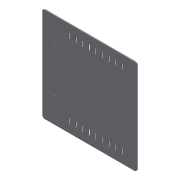
# Autodesk Inventor part: Plate A for Power Boards
Saved by Autodesk Inventor 2015 (Build 190159000, 159)
## iProperties
Created: 2015-01-10
Part Number: Plate A for Power Boards
Material: Generic
Document SubType Name: Sheet Metal
Designer: Peter
Density: 1 g/cm^3
Sheet Metal Rule: Default
Appearance: Default
Author: Peter
Autodesk Inventor part; units mm, degrees
ref_plane "YZ Plane" through (0, 0, 0) normal (1, 0, 0) x (0, 1, 0)
sketch "Sketch1" plane through (0, 0, 0) normal (0, 0, 1) x (1, 0, 0)
  line L0 (0, 0) -> (228.6, 0)
  line L1 (228.6, 0) -> (228.6, 228.6)
  line L2 (228.6, 228.6) -> (0, 228.6)
  line L3 (0, 228.6) -> (0, 0)
  dimension "d0" = 228.6
  dimension "d1" = 228.6
  measures "d0" distance of L2.end L1.end
  measures "d1" distance of L1.end L0.end
extrude "Plate1" add sketch "Sketch1" along normal blind 2.286
ref_plane "Work Plane1" through (114.3, 0, 0) normal (1, 0, 0) x (0, 0, -1)
ref_plane "Work Plane2" through (0, 114.3, 0) normal (0, 1, 0) x (1, 0, 0)
sketch "Sketch2" plane through (0, 0, 2.286) normal (0, 0, 1) x (1, 0, 0)
  circle A0 centre (29.3437, 62.0361) radius 2.667 projected
  circle A1 centre (29.3437, 166.4301) radius 2.667 projected
  circle A2 centre (211.6141, 166.4301) radius 2.667 projected
  circle A3 centre (211.6141, 62.0361) radius 2.667 projected
  circle A4 centre (29.3437, 62.0361) radius 1.5875
  circle A5 centre (29.3437, 166.4301) radius 1.5875
  circle A6 centre (211.6141, 166.4301) radius 1.5875
  circle A7 centre (211.6141, 62.0361) radius 1.5875
  dimension "x" = 3.175
  dimension "d5" = 3.175
  dimension "d6" = 3.175
  dimension "d7" = 3.175
  constraints: 4 centre point, 4 coincident
  measures "x" diameter of A4
  measures "d5" diameter of A5
  measures "d6" diameter of A6
  measures "d7" diameter of A7
sketch "Sketch3" plane through (0, 0, 2.286) normal (0, 0, 1) x (1, 0, 0)
  line L0 (0, 0) -> (0, 228.6) projected
  line L1 (228.6, 0) -> (0, 0) projected
  line L2 (228.6, 228.6) -> (228.6, 0) projected
  line L3 (0, 228.6) -> (228.6, 228.6) projected
hole "Hole1" at (29.3437, 62.0361, 2.286) direction (0, 0, -1) diameter 3.175 end through all
hole "Hole2" at (211.6141, 62.0361, 2.286) direction (0, 0, -1) diameter 3.175 end through all
hole "Hole3" at (211.6141, 166.4301, 2.286) direction (0, 0, -1) diameter 3.175 end through all
hole "Hole4" at (29.3437, 166.4301, 2.286) direction (0, 0, -1) diameter 3.175 end through all
sketch "Sketch4" plane through (0, 0, 2.286) normal (0, 0, 1) x (1, 0, 0)
  line L0 (0, 228.6) -> (228.6, 228.6) projected
  line L1 (63.5, 196.85) -> (66.675, 196.85)
  line L2 (66.675, 196.85) -> (66.675, 209.55)
  line L3 (66.675, 209.55) -> (63.5, 209.55)
  line L4 (63.5, 209.55) -> (63.5, 196.85)
  line L5 (79.375, 196.85) -> (82.55, 196.85)
  line L6 (82.55, 196.85) -> (82.55, 209.55)
  line L7 (82.55, 209.55) -> (79.375, 209.55)
  line L8 (79.375, 209.55) -> (79.375, 196.85)
  line L9 (95.25, 196.85) -> (98.425, 196.85)
  line L10 (98.425, 196.85) -> (98.425, 209.55)
  line L11 (98.425, 209.55) -> (95.25, 209.55)
  line L12 (95.25, 209.55) -> (95.25, 196.85)
  line L13 (111.125, 196.85) -> (114.3, 196.85)
  line L14 (114.3, 196.85) -> (114.3, 209.55)
  line L15 (114.3, 209.55) -> (111.125, 209.55)
  line L16 (111.125, 209.55) -> (111.125, 196.85)
  line L17 (127, 196.85) -> (130.175, 196.85)
  line L18 (130.175, 196.85) -> (130.175, 209.55)
  line L19 (130.175, 209.55) -> (127, 209.55)
  line L20 (127, 209.55) -> (127, 196.85)
  line L21 (142.875, 196.85) -> (146.05, 196.85)
  line L22 (146.05, 196.85) -> (146.05, 209.55)
  line L23 (146.05, 209.55) -> (142.875, 209.55)
  line L24 (142.875, 209.55) -> (142.875, 196.85)
  line L25 (158.75, 196.85) -> (161.925, 196.85)
  line L26 (161.925, 196.85) -> (161.925, 209.55)
  line L27 (161.925, 209.55) -> (158.75, 209.55)
  line L28 (158.75, 209.55) -> (158.75, 196.85)
  line L29 (174.625, 196.85) -> (177.8, 196.85)
  line L30 (177.8, 196.85) -> (177.8, 209.55)
  line L31 (177.8, 209.55) -> (174.625, 209.55)
  line L32 (174.625, 209.55) -> (174.625, 196.85)
  line L33 (190.5, 196.85) -> (193.675, 196.85)
  line L34 (193.675, 196.85) -> (193.675, 209.55)
  line L35 (193.675, 209.55) -> (190.5, 209.55)
  line L36 (190.5, 209.55) -> (190.5, 196.85)
  dimension "d36" = 12.7
  dimension "d37" = 3.175
  dimension "d38" = 19.05
  dimension "d39" = 63.5
  dimension "d42" = 15.875
  constraints: 72 end point, 2 horizontal, 2 parallel, 1 perpendicular, 64 other
  measures "d36" distance of L3.end L1.start
  measures "d37" distance of L1.start L1.end
  measures "d38" vertical distance of L3.end L0.start
  measures "d39" horizontal distance of L0.start L3.end
  measures "d42" distance of L3.end L8.start
extrude "Cut1" cut sketch "Sketch4" against normal blind 2.286
mirror "Mirror1" about plane through (0, 114.3, 0) normal (0, 1, 0) of "Cut1"
fillet "Corner Round1" radius 6.35 1 edges at (228.6, 228.6, 1.143)
fillet "Corner Round2" radius 6.35 3 edges at (228.6, 0, 1.143) (0, 0, 1.143) (0, 228.6, 1.143)
equation "\"d5\" = x"
equation "\"d6\" = x"
equation "\"d7\" = x"
equation "\"d13\" = Thickness"
equation "\"d20\" = Thickness"
equation "\"d27\" = Thickness"
equation "\"d34\" = Thickness"
equation "\"d47\" = Thickness"
equation "\"BendRadius\" = Thickness"
equation "\"BendReliefWidth\" = Thickness"
equation "\"BendReliefDepth\" = 0.5 * Thickness"
equation "\"CornerReliefSize\" = 4 * Thickness"
equation "\"MinimumRemnant\" = 2 * Thickness"
equation "\"TransitionRadius\" = BendRadius"
equation "\"JacobiRadiusSize\" = BendRadius"
equation "\"GapSize\" = Thickness"
equation "\"d2\" = BendRadius"
equation "\"Thickness\" = 2.286"
body "Solid1"
